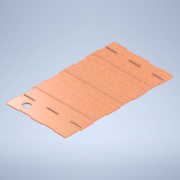
# Autodesk Inventor part: Rear_V2
Saved by Autodesk Inventor 2022.2 (Build 262287000, 287)
## iProperties
Created: 2022-11-15
Part Number: Rear_V2
Material: Generic
Document SubType Name: Modeling
Designer: jaege
Density: 1 g/cm^3
Appearance: Red Oak - Natural Low Gloss
Mass: 450.623 g
Surface Area: 2376.39 cm^2
Volume: 450.623 cm^3
Author: jaege
Autodesk Inventor part; units mm, degrees
ref_plane "YZ Plane" through (0, 0, 0) normal (1, 0, 0) x (0, 1, 0)
ref_plane "XZ Plane" through (0, 0, 0) normal (0, 1, 0) x (-1, 0, 0)
ref_plane "XY Plane" through (0, 0, 0) normal (0, 0, 1) x (1, 0, 0)
sketch "Sketch1" plane through (0, 0, 0) normal (0, 1, 0) x (-1, 0, 0)
  line L0 (-125, 225) -> (125, 225) construction
  line L1 (125, 225) -> (125, -225) construction
  line L2 (125, -225) -> (-125, -225) construction
  line L3 (-125, -225) -> (-125, 225) construction
  line L4 (-125, 225) -> (125, -225) construction
  line L5 (125, 225) -> (-125, -225) construction
  line L6 (125, 225) -> (75, 225) construction
  line L7 (75, 225) -> (75, 229)
  line L8 (75, 229) -> (125, 229)
  line L9 (125, 229) -> (125, 225)
  line L10 (125, 225) -> (129, 225)
  line L11 (129, 225) -> (129, 168.75)
  line L12 (129, 168.75) -> (125, 168.75)
  line L13 (125, 168.75) -> (125, 225) construction
  line L14 (-125, 225) -> (-129, 225) construction
  line L15 (-129, 225) -> (-129, 168.75) construction
  line L16 (-129, 168.75) -> (-125, 168.75)
  line L17 (-125, 168.75) -> (-125, 225)
  line L18 (125, -225) -> (75, -225) construction
  line L19 (75, -225) -> (75, -229)
  line L20 (75, -229) -> (125, -229)
  line L21 (125, -229) -> (125, -225)
  line L22 (125, 112.5) -> (125, 168.75)
  line L23 (125, 168.75) -> (129, 168.75)
  line L24 (129, 112.5) -> (125, 112.5)
  line L25 (129, 168.75) -> (129, 112.5) construction
  line L26 (-125, 112.5) -> (-125, 168.75) construction
  line L27 (-125, 168.75) -> (-129, 168.75)
  line L28 (-129, 168.75) -> (-129, 112.5)
  line L29 (-129, 112.5) -> (-125, 112.5)
  line L30 (125, 56.25) -> (125, 112.5) construction
  line L31 (125, 112.5) -> (129, 112.5)
  line L32 (129, 56.25) -> (125, 56.25)
  line L33 (129, 112.5) -> (129, 56.25)
  line L34 (-125, 56.25) -> (-125, 112.5)
  line L35 (-125, 112.5) -> (-129, 112.5)
  line L36 (-129, 112.5) -> (-129, 56.25) construction
  line L37 (-129, 56.25) -> (-125, 56.25)
  line L38 (125, 0) -> (125, 56.25)
  line L39 (125, 56.25) -> (129, 56.25)
  line L40 (129, 0) -> (125, 0)
  line L41 (129, 56.25) -> (129, 0) construction
  line L42 (-125, 0) -> (-125, 56.25) construction
  line L43 (-125, 56.25) -> (-129, 56.25)
  line L44 (-129, 56.25) -> (-129, 0)
  line L45 (-129, 0) -> (-125, 0)
  line L46 (125, -56.25) -> (125, 0) construction
  line L47 (125, 0) -> (129, 0)
  line L48 (129, -56.25) -> (125, -56.25)
  line L49 (129, 0) -> (129, -56.25)
  line L50 (-125, -56.25) -> (-125, 0)
  line L51 (-125, 0) -> (-129, 0)
  line L52 (-129, 0) -> (-129, -56.25) construction
  line L53 (-129, -56.25) -> (-125, -56.25)
  line L54 (125, -112.5) -> (125, -56.25)
  line L55 (125, -56.25) -> (129, -56.25)
  line L56 (129, -112.5) -> (125, -112.5)
  line L57 (129, -56.25) -> (129, -112.5) construction
  line L58 (-125, -112.5) -> (-125, -56.25) construction
  line L59 (-125, -56.25) -> (-129, -56.25)
  line L60 (-129, -56.25) -> (-129, -112.5)
  line L61 (-129, -112.5) -> (-125, -112.5)
  line L62 (125, -168.75) -> (125, -112.5) construction
  line L63 (125, -112.5) -> (129, -112.5)
  line L64 (129, -168.75) -> (125, -168.75)
  line L65 (129, -112.5) -> (129, -168.75)
  line L66 (-125, -168.75) -> (-125, -112.5)
  line L67 (-125, -112.5) -> (-129, -112.5)
  line L68 (-129, -112.5) -> (-129, -168.75) construction
  line L69 (-129, -168.75) -> (-125, -168.75)
  line L70 (125, -225) -> (125, -168.75)
  line L71 (125, -168.75) -> (129, -168.75)
  line L72 (129, -225) -> (125, -225) construction
  line L73 (129, -168.75) -> (129, -225) construction
  line L74 (-125, -225) -> (-125, -168.75) construction
  line L75 (-125, -168.75) -> (-129, -168.75)
  line L76 (-129, -168.75) -> (-129, -225)
  line L77 (-129, -225) -> (-125, -225)
  line L78 (75, 229) -> (75, 225)
  line L79 (25, 225) -> (25, 229)
  line L80 (25, 229) -> (75, 229) construction
  line L81 (75, 225) -> (25, 225)
  line L82 (75, -225) -> (25, -225)
  line L83 (25, -225) -> (25, -229)
  line L84 (25, -229) -> (75, -229) construction
  line L85 (75, -229) -> (75, -225)
  line L86 (25, 229) -> (25, 225)
  line L87 (-25, 225) -> (-25, 229)
  line L88 (-25, 229) -> (25, 229)
  line L89 (25, 225) -> (-25, 225) construction
  line L90 (25, -225) -> (-25, -225) construction
  line L91 (-25, -225) -> (-25, -229)
  line L92 (-25, -229) -> (25, -229)
  line L93 (25, -229) -> (25, -225)
  line L94 (-25, 229) -> (-25, 225)
  line L95 (-75, 225) -> (-75, 229)
  line L96 (-75, 229) -> (-25, 229) construction
  line L97 (-25, 225) -> (-75, 225)
  line L98 (-25, -225) -> (-75, -225)
  line L99 (-75, -225) -> (-75, -229)
  line L100 (-75, -229) -> (-25, -229) construction
  line L101 (-25, -229) -> (-25, -225)
  line L102 (-75, 229) -> (-75, 225)
  line L103 (-125, 225) -> (-125, 229)
  line L104 (-125, 229) -> (-75, 229)
  line L105 (-75, 225) -> (-125, 225) construction
  line L106 (-75, -225) -> (-125, -225) construction
  line L107 (-125, -225) -> (-125, -229)
  line L108 (-125, -229) -> (-75, -229)
  line L109 (-75, -229) -> (-75, -225)
  point P0 (0, 0)
  point P1 (75, -225)
  point P2 (25, -225)
  point P3 (-25, -225)
  point P4 (-75, -225)
  point P5 (-129, 168.75)
  point P6 (-129, 56.25)
  point P7 (-129, -56.25)
  point P8 (-129, -168.75)
  point P9 (-125, -225)
  point P10 (-25, -225)
  point P11 (75, -225)
  point P12 (125, -56.25)
  point P13 (125, 56.25)
  point P14 (125, 168.75)
  dimension "d0" = 250
  dimension "d1" = 450
  dimension "d2" = 50
  dimension "d3" = 4
  dimension "d4" = 4
  dimension "d5" = 56.25
  dimension "d6" = 4
  dimension "d7" = 56.25
  dimension "d8" = 50
  dimension "d9" = 4
  dimension "d12" = 56.25
  dimension "d19" = 50
  constraints: 220 end point, 10 parallel, 6 horizontal, 5 perpendicular, 2 midpoint, 1 vertical, 180 other
  measures "d0" distance of L1.end L2.end
  measures "d1" distance of L0.end L1.end
  measures "d2" distance of L7.end L8.end
  measures "d3" distance of L6.end L7.end
  measures "d4" distance of L11.end L12.end
  measures "d5" distance of L10.end L11.end
  measures "d6" distance of L16.end L15.end
  measures "d7" distance of L15.end L14.end
  measures "d8" distance of L20.end L19.end
  measures "d9" distance of L19.end L18.end
  measures "d12" distance of L0.end L22.end
  measures "d19" distance of L0.end L78.end
extrude "Extrusion1" add sketch "Sketch1" along normal blind 4
sketch "Sketch3" plane through (0, 4, 0) normal (0, 1, 0) x (1, 0, 0)
  line L0 (-129, 56.25) -> (-129, 0) projected
  line L1 (-129, 15.625) -> (125, 15.625) construction
  line L2 (125, 0) -> (125, 56.25) projected
  line L3 (-129, 13.125) -> (125, 13.125)
  line L4 (125, 13.125) -> (125, 18.125)
  line L5 (125, 18.125) -> (-129, 18.125)
  line L6 (-129, 18.125) -> (-129, 13.125)
  line L7 (-129, 18.125) -> (-125, 18.125)
  line L8 (-125, 18.125) -> (-125, 13.125)
  line L9 (-125, 13.125) -> (-129, 13.125)
  line L10 (-129, 13.125) -> (-129, 18.125)
  line L11 (-25, -225) -> (-25, -229) projected
  line L12 (-25, -229) -> (25, -229) projected
  line L13 (25, -229) -> (25, -225) projected
  line L14 (25, -225) -> (75, -225) projected
  line L15 (75, -225) -> (75, -229) projected
  line L16 (75, -229) -> (125, -229) projected
  line L17 (125, -229) -> (125, -168.75) projected
  line L18 (125, -168.75) -> (129, -168.75) projected
  line L19 (129, -168.75) -> (129, -112.5) projected
  line L20 (129, -112.5) -> (125, -112.5) projected
  line L21 (125, -112.5) -> (125, -56.25) projected
  line L22 (125, -56.25) -> (129, -56.25) projected
  line L23 (129, -56.25) -> (129, 0) projected
  line L24 (129, 0) -> (125, 0) projected
  line L25 (125, 0) -> (125, 56.25) projected
  line L26 (125, 56.25) -> (129, 56.25) projected
  line L27 (129, 56.25) -> (129, 112.5) projected
  line L28 (129, 112.5) -> (125, 112.5) projected
  line L29 (125, 112.5) -> (125, 168.75) projected
  line L30 (125, 168.75) -> (129, 168.75) projected
  line L31 (129, 168.75) -> (129, 225) projected
  line L32 (129, 225) -> (125, 225) projected
  line L33 (125, 225) -> (125, 229) projected
  line L34 (125, 229) -> (75, 229) projected
  line L35 (75, 229) -> (75, 225) projected
  line L36 (75, 225) -> (25, 225) projected
  line L37 (25, 225) -> (25, 229) projected
  line L38 (25, 229) -> (-25, 229) projected
  line L39 (-25, 229) -> (-25, 225) projected
  line L40 (-25, 225) -> (-75, 225) projected
  line L41 (-75, 225) -> (-75, 229) projected
  line L42 (-75, 229) -> (-125, 229) projected
  line L43 (-125, 229) -> (-125, 168.75) projected
  line L44 (-125, 168.75) -> (-129, 168.75) projected
  line L45 (-129, 168.75) -> (-129, 112.5) projected
  line L46 (-129, 112.5) -> (-125, 112.5) projected
  line L47 (-125, 112.5) -> (-125, 56.25) projected
  line L48 (-125, 56.25) -> (-129, 56.25) projected
  line L49 (-129, 56.25) -> (-129, 0) projected
  line L50 (-129, 0) -> (-125, 0) projected
  line L51 (-125, 0) -> (-125, -56.25) projected
  line L52 (-125, -56.25) -> (-129, -56.25) projected
  line L53 (-129, -56.25) -> (-129, -112.5) projected
  line L54 (-129, -112.5) -> (-125, -112.5) projected
  line L55 (-125, -112.5) -> (-125, -168.75) projected
  line L56 (-125, -168.75) -> (-129, -168.75) projected
  line L57 (-129, -168.75) -> (-129, -225) projected
  line L58 (-129, -225) -> (-125, -225) projected
  line L59 (-125, -225) -> (-125, -229) projected
  line L60 (-125, -229) -> (-75, -229) projected
  line L61 (-75, -229) -> (-75, -225) projected
  line L62 (-75, -225) -> (-25, -225) projected
  line L63 (-125, -112.5) -> (-125, -168.75) projected
  line L64 (-109.8402, -80.4521) -> (129, -140.625) construction
  line L65 (129, -168.75) -> (129, -112.5) projected
  line L66 (-125, -110.625) -> (125, -110.625)
  line L67 (125, -110.625) -> (125, -105.625)
  line L68 (125, -105.625) -> (-125, -105.625)
  line L69 (-125, -105.625) -> (-125, -110.625)
  line L70 (-125, -110.625) -> (125, -105.625) construction
  line L71 (125, -110.625) -> (-125, -105.625) construction
  line L72 (125, 0) -> (125, 56.25) projected
  line L73 (-125, 0) -> (-125, -56.25) projected
  line L74 (129, 168.75) -> (129, 225) projected
  line L75 (129, 139.375) -> (-125, 139.375) construction
  line L76 (-125, 136.875) -> (125, 136.875)
  line L77 (125, 136.875) -> (125, 141.875)
  line L78 (125, 141.875) -> (-125, 141.875)
  line L79 (-125, 141.875) -> (-125, 136.875)
  line L80 (-125, 136.875) -> (125, 141.875) construction
  line L81 (125, 136.875) -> (-125, 141.875) construction
  line L82 (-125, 229) -> (-125, 168.75) projected
  line L83 (125, 112.5) -> (125, 168.75) projected
  point P0 (0, 0)
  point P1 (-129, 18.125)
  point P2 (-125, 18.125)
  point P3 (-125, 13.125)
  point P4 (0, -108.125)
  point P5 (-125, -138.125)
  point P6 (-125, -143.125)
  point P7 (0, 139.375)
  point P8 (-125, 199.375)
  point P9 (-125, 194.375)
  dimension "d30" = 5
  dimension "d34" = 5
  dimension "d35" = 5
  dimension "d36" = 5
  dimension "d56" = 118.375
  dimension "d57" = 118.75
  dimension "d59" = 118.75
  constraints: 46 end point, 8 parallel, 5 collinear, 5 midpoint, 5 perpendicular, 4 horizontal, 4 point on line, 1 other
  measures "d30" distance of L4.end L3.end
  measures "d34" distance of L7.end L8.end
  measures "d35" distance of L66.end L67.end
  measures "d36" distance of L76.end L77.end
  measures "d56" distance between parallel lines of L60 L66
  measures "d57" distance between parallel lines of L68 L3
  measures "d59" distance between parallel lines of L5 L76
extrude "Extrusion2" cut sketch "Sketch3" against normal blind 1 contours L5 L2 L3 L8 | L76 L79 L78 L29 | L21 L66 L69 L68
sketch "Sketch4" plane through (0, 4, 0) normal (0, 1, 0) x (1, 0, 0)
  line L0 (-125, -158) -> (-75, -158)
  line L1 (-75, -158) -> (-75, -162)
  line L2 (-75, -162) -> (-125, -162)
  line L3 (-125, -162) -> (-125, -158)
  line L4 (-75, -225) -> (-25, -225) projected
  line L5 (125, -110.625) -> (-125, -110.625) projected
  line L6 (-75, -158) -> (-25, -158)
  line L7 (-25, -158) -> (-25, -162)
  line L8 (-25, -162) -> (-75, -162)
  line L9 (-75, -162) -> (-75, -158)
  line L10 (-25, -158) -> (25, -158)
  line L11 (25, -158) -> (25, -162)
  line L12 (25, -162) -> (-25, -162)
  line L13 (-25, -162) -> (-25, -158)
  line L14 (25, -158) -> (75, -158)
  line L15 (75, -158) -> (75, -162)
  line L16 (75, -162) -> (25, -162)
  line L17 (25, -162) -> (25, -158)
  line L18 (75, -158) -> (125, -158)
  line L19 (125, -158) -> (125, -162)
  line L20 (125, -162) -> (75, -162)
  line L21 (75, -162) -> (75, -158)
  line L22 (-125, 0) -> (-125, -56.25) projected
  line L23 (-125, 192) -> (-75, 192)
  line L24 (-75, 192) -> (-75, 188)
  line L25 (-75, 188) -> (-125, 188)
  line L26 (-125, 188) -> (-125, 192)
  line L27 (-75, 192) -> (-25, 192)
  line L28 (-25, 192) -> (-25, 188)
  line L29 (-25, 188) -> (-25, 192)
  line L30 (-25, 188) -> (-75, 188)
  line L31 (-75, 188) -> (-75, 192)
  line L32 (-25, 192) -> (25, 192)
  line L33 (25, 188) -> (-25, 188)
  line L34 (25, 192) -> (25, 188)
  line L35 (25, 188) -> (25, 192)
  line L36 (25, 192) -> (75, 192)
  line L37 (75, 192) -> (75, 188)
  line L38 (75, 188) -> (75, 192)
  line L39 (75, 192) -> (125, 192)
  line L40 (125, 192) -> (125, 188)
  line L41 (125, 188) -> (75, 188)
  line L42 (75, 188) -> (25, 188)
  point P0 (0, 0)
  point P1 (-125, -160)
  point P2 (-75, -160)
  point P3 (-25, -160)
  point P4 (25, -160)
  point P5 (75, -160)
  point P6 (-25, -162)
  point P7 (-125, 190)
  point P8 (-25, 190)
  point P9 (-75, 190)
  point P10 (25, 190)
  point P11 (75, 190)
  point P12 (-25, 188)
  point P13 (-125, -168.75)
  dimension "d37" = 50
  dimension "d38" = 4
  dimension "d39" = 63
  dimension "d42" = 50
  dimension "d51" = 350
  constraints: 80 end point, 2 horizontal, 2 parallel, 1 midpoint, 1 perpendicular, 1 vertical, 1 vertical alignment, 81 other
  measures "d37" distance of L1.end L2.end
  measures "d38" distance of L0.end L1.end
  measures "d39" distance between parallel lines of L4 L2
  measures "d42" distance of L0.start L6.start
  measures "d51" distance of L0.start L23.start
extrude "Extrusion3" cut sketch "Sketch4" against normal up to next contours L0 L1 L2 L3 | L10 L11 L12 L7 | L18 L19 L20 L15 | L23 L24 L25 L26 | L32 L34 L33 L28 | L39 L40 L41 L37
sketch "Sketch6" plane through (0, 4, 0) normal (0, 1, 0) x (1, 0, 0)
  circle A0 centre (-75, -195) radius 15
  line L0 (-75, -225) -> (-25, -225) projected
  line L1 (-125, -162) -> (-125, -168.75) projected
  point P0 (0, 0)
  point P1 (-125, -165.375)
  dimension "d60" = 30
  dimension "d61" = 30
  dimension "d62" = 50
  constraints: 1 centre point, 1 midpoint
  measures "d60" diameter of A0
  measures "d61" distance from line of L0 A0.centre
  measures "d62" horizontal distance of point (-125, -165.375) A0.centre
extrude "Extrusion4" cut sketch "Sketch6" against normal through all
body "Solid1"
